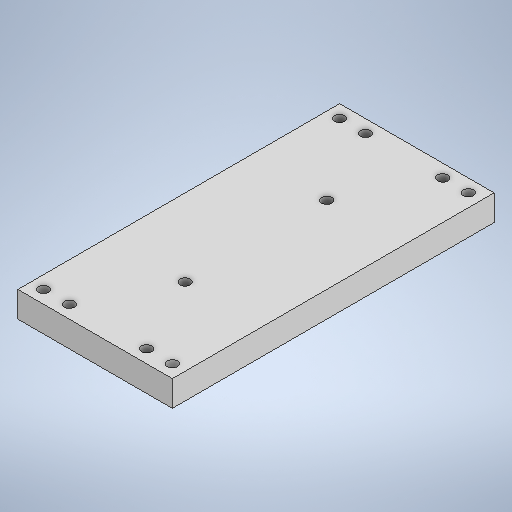
# Autodesk Inventor part: Rb PEEK - Arriba
Saved by Autodesk Inventor 2025.3 (Build 293356000, 356)
## iProperties
Created: 2025-05-09
Part Number: Rb PEEK - Arriba
Material: Generic
Document SubType Name: Modeling
Designer: E. Moreno
Density: 1 g/cm^3
Appearance: Default
Title: Rb PEEK - Abajo
Author: E. Moreno
Autodesk Inventor part; units mm, degrees
ref_plane "YZ Plane" through (0, 0, 0) normal (1, 0, 0) x (0, 1, 0)
ref_plane "XZ Plane" through (0, 0, 0) normal (0, 1, 0) x (-1, 0, 0)
ref_plane "XY Plane" through (0, 0, 0) normal (0, 0, 1) x (1, 0, 0)
sketch "Sketch1" plane through (0, 0, 0) normal (0, 1, 0) x (-1, 0, 0)
  line L0 (-30, 62.5) -> (30, 62.5)
  line L1 (30, 62.5) -> (30, -62.5)
  line L2 (30, -62.5) -> (-30, -62.5)
  line L3 (-30, -62.5) -> (-30, 62.5)
  line L4 (-30, 62.5) -> (30, -62.5) construction
  line L5 (30, 62.5) -> (-30, -62.5) construction
  point P0 (0, 0)
  dimension "d0" = 60
  dimension "d1" = 125
  constraints: 12 end point, 2 midpoint, 2 parallel, 1 horizontal, 1 perpendicular
  measures "d0" distance of L1.end L2.end
  measures "d1" distance of L0.end L1.end
extrude "Extrusion1" add sketch "Sketch1" along normal blind 10
sketch "Sketch2" plane through (0, 10, 0) normal (0, 1, 0) x (1, 0, 0)
  line L0 (-30, -62.5) -> (30, -62.5) projected
  line L1 (30, -62.5) -> (30, -57.5)
  line L2 (30, -62.5) -> (30, 62.5) projected
  line L3 (30, -57.5) -> (25, -57.5)
  circle A0 centre (25, -57.5) radius 2
  line L4 (25, -57.5) -> (15, -57.5)
  circle A1 centre (15, -57.5) radius 2
  line L5 (0, 0) -> (30, 0)
  line L6 (-30, 62.5) -> (30, 62.5)
  line L7 (30, 62.5) -> (30, 57.5)
  line L8 (30, 62.5) -> (30, -62.5)
  line L9 (30, 57.5) -> (25, 57.5)
  circle A2 centre (25, 57.5) radius 2
  line L10 (25, 57.5) -> (15, 57.5)
  circle A3 centre (15, 57.5) radius 2
  line L11 (0, -62.5) -> (0, 62.5)
  line L12 (-30, -62.5) -> (-30, -57.5)
  line L13 (-30, -62.5) -> (-30, 62.5)
  line L14 (-30, -57.5) -> (-25, -57.5)
  circle A4 centre (-25, -57.5) radius 2
  line L15 (-25, -57.5) -> (-15, -57.5)
  circle A5 centre (-15, -57.5) radius 2
  line L16 (-30, 62.5) -> (-30, 57.5)
  line L17 (-30, 62.5) -> (-30, -62.5)
  line L18 (-30, 57.5) -> (-25, 57.5)
  circle A6 centre (-25, 57.5) radius 2
  line L19 (-25, 57.5) -> (-15, 57.5)
  circle A7 centre (-15, 57.5) radius 2
  point P0 (-30, 0)
  dimension "d4" = 5
  dimension "d5" = 5
  dimension "d6" = 4
  dimension "d7" = 10
  dimension "d8" = 4
  constraints: 36 end point, 23 symmetric about line, 8 centre point, 8 coincident, 4 point on line, 3 midpoint, 2 horizontal, 6 other
  measures "d4" distance of L0.end L1.end
  measures "d5" distance of L1.end L3.end
  measures "d6" diameter of A0
  measures "d7" distance of L4.start L4.end
  measures "d8" diameter of A1
extrude "Extrusion2" cut sketch "Sketch2" against normal blind 10 contours A0 L4 L3 | L3 L4 A0 | A1 | A2 L10 L9 | L9 L10 A2 | A3 | A4 L15 L14 | L14 L15 A4 | A5 | A6 L19 L18 | L18 L19 A6 | A7
sketch "Sketch3" plane through (0, 10, 0) normal (0, 1, 0) x (1, 0, 0)
  circle A0 centre (25, -57.5) radius 3.61
  circle A1 centre (25, -57.5) radius 2 projected
  circle A2 centre (15, -57.5) radius 3.61
  circle A3 centre (15, -57.5) radius 2 projected
  line L0 (0, 0) -> (29.9913, 0)
  line L1 (-30, -62.5) -> (30, -62.5) projected
  line L2 (0, -62.5) -> (0, 62.5)
  line L3 (30, 62.5) -> (-30, 62.5) projected
  circle A4 centre (15, -57.5) radius 2
  circle A5 centre (25, -57.5) radius 2
  circle A6 centre (25, 57.5) radius 3.61
  circle A7 centre (25, 57.5) radius 2
  circle A8 centre (15, 57.5) radius 3.61
  circle A9 centre (15, 57.5) radius 2
  circle A10 centre (15, 57.5) radius 2
  circle A11 centre (25, 57.5) radius 2
  circle A12 centre (-25, -57.5) radius 3.61
  circle A13 centre (-25, -57.5) radius 2
  circle A14 centre (-15, -57.5) radius 3.61
  circle A15 centre (-15, -57.5) radius 2
  circle A16 centre (-15, -57.5) radius 2
  circle A17 centre (-25, -57.5) radius 2
  circle A18 centre (-25, 57.5) radius 3.61
  circle A19 centre (-25, 57.5) radius 2
  circle A20 centre (-15, 57.5) radius 3.61
  circle A21 centre (-15, 57.5) radius 2
  circle A22 centre (-15, 57.5) radius 2
  circle A23 centre (-25, 57.5) radius 2
  point P0 (-29.9913, 0)
  dimension "d11" = 7.22
  dimension "d12" = 7.22
  dimension "d13" = 4
  dimension "d14" = 4
  constraints: 22 centre point, 19 symmetric about line, 4 concentric, 4 end point, 2 midpoint, 1 horizontal, 18 other
  measures "d11" diameter of A0
  measures "d12" diameter of A2
  measures "d13" diameter of A4
  measures "d14" diameter of A5
extrude "Extrusion3" cut sketch "Sketch3" against normal blind 4.5
sketch "Sketch6" plane through (0, 10, 0) normal (0, 1, 0) x (1, 0, 0)
  line L0 (-30, -62.5) -> (30, -62.5) projected
  line L1 (-30, -62.5) -> (0, -62.5)
  line L2 (0, -62.5) -> (0, -27.5)
  circle A0 centre (0, -27.5) radius 2
  line L3 (-30, 62.5) -> (-30, -62.5) projected
  line L4 (-30, 0) -> (30, 0)
  line L5 (30, -62.5) -> (30, 62.5) projected
  circle A1 centre (0, 27.5) radius 2
  point P0 (0, 0)
  dimension "d24" = 35
  dimension "d25" = 4
  constraints: 6 end point, 3 midpoint, 2 centre point, 2 coincident, 2 symmetric about line, 1 vertical, 1 other
  measures "d24" distance of L1.end L2.end
  measures "d25" diameter of A0
extrude "Extrusion6" cut sketch "Sketch6" against normal blind 10 contours A0 | A1
sketch "Sketch7" plane through (0, 10, 0) normal (0, 1, 0) x (1, 0, 0)
  circle A0 centre (0, -27.5) radius 3.61
  circle A1 centre (0, -27.5) radius 2 projected
  line L0 (-30, 62.5) -> (-30, -62.5) projected
  line L1 (-30, 0) -> (30, 0)
  line L2 (30, -62.5) -> (30, 62.5) projected
  circle A2 centre (0, 27.5) radius 3.61
  circle A3 centre (0, 27.5) radius 2
  point P0 (0, 0)
  dimension "d28" = 7.22
  constraints: 3 centre point, 2 end point, 2 midpoint, 2 symmetric about line, 1 concentric, 2 other
  measures "d28" diameter of A0
extrude "Extrusion7" cut sketch "Sketch7" against normal blind 4.5
mirror "Mirror1" about plane through (0, 0, 0) normal (0, 1, 0) remove original yes
body "Solid1"
